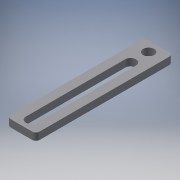
# Autodesk Inventor part: ButtonLockerV2
Saved by Autodesk Inventor 2018 (Build 220112000, 112)
## iProperties
Created: 2018-05-22
Part Number: ButtonLockerV2
Material: Generic
Document SubType Name: Modeling
Designer: reide
Density: 1 g/cm^3
Appearance: Default
Author: reide
Autodesk Inventor part; units mm, degrees
ref_plane "YZ Plane" through (0, 0, 0) normal (1, 0, 0) x (0, 1, 0)
ref_plane "XZ Plane" through (0, 0, 0) normal (0, 1, 0) x (-1, 0, 0)
ref_plane "XY Plane" through (0, 0, 0) normal (0, 0, 1) x (1, 0, 0)
sketch "Sketch1" plane through (0, 0, 0) normal (0, 0, 1) x (1, 0, 0)
  line L0 (35.2961, 108.9853) -> (93.2961, 108.9853)
  line L1 (35.2961, 103.4853) -> (35.2961, 108.9853)
  line L2 (93.2961, 103.4853) -> (35.2961, 103.4853)
  line L3 (93.2961, 108.9853) -> (93.2961, 103.4853)
  line L4 (2, 88) -> (126.0922, 88)
  line L5 (2, 80) -> (2, 88)
  line L6 (2, 80) -> (126.0922, 80)
  line L7 (126.0922, 80) -> (126.0922, 88)
  line L8 (11.7071, 1) -> (2, 1)
  line L9 (11.7071, 80) -> (11.7071, 1)
  line L10 (2, 80) -> (11.7071, 80)
  line L11 (2, 1) -> (2, 80)
  line L12 (126.0922, 80) -> (126.0922, 1)
  line L13 (126.0922, 1) -> (116.3851, 1)
  line L14 (126.0922, 80) -> (126.0922, 1)
  line L15 (116.3851, 80) -> (126.0922, 80)
  line L16 (116.3851, 1) -> (116.3851, 80)
  line L17 (102.7961, 70.9853) -> (96.2961, 70.9853)
  line L18 (102.7961, 108.9853) -> (102.7961, 70.9853)
  line L19 (95.2961, 108.9853) -> (102.7961, 108.9853)
  line L20 (95.2961, 103.4853) -> (95.2961, 108.9853)
  line L21 (96.2961, 103.4853) -> (95.2961, 103.4853)
  line L22 (96.2961, 103.4853) -> (96.2961, 70.9853)
  line L23 (32.2961, 70.9853) -> (25.7961, 70.9853)
  line L24 (32.2961, 103.4853) -> (32.2961, 70.9853)
  line L25 (33.2961, 103.4853) -> (32.2961, 103.4853)
  line L26 (33.2961, 108.9853) -> (33.2961, 103.4853)
  line L27 (25.7961, 108.9853) -> (33.2961, 108.9853)
  line L28 (25.7961, 70.9853) -> (25.7961, 108.9853)
  line L29 (64.2961, 108.9853) -> (64.2961, 70.9853)
  line L30 (64.2961, 108.9853) -> (68.2961, 108.9853)
  line L31 (68.2961, 108.9853) -> (60.2961, 108.9853)
  line L32 (60.2961, 108.9853) -> (66.2961, 108.9853)
  line L33 (66.2961, 70.4263) -> (60.2961, 70.4263)
  line L34 (60.2961, 70.4263) -> (60.2961, 108.9853)
  circle A0 centre (64.2961, 106.2353) radius 1.75
  line L35 (68.2961, 108.9853) -> (60.2961, 108.9853)
  line L36 (60.2961, 108.9853) -> (60.2961, 70.4263)
  line L37 (60.2961, 70.4263) -> (68.2961, 70.4263)
  line L38 (68.2961, 70.4263) -> (68.2961, 108.9853)
  line L39 (64.2961, 106.2353) -> (64.2961, 101.2353)
  line L40 (68.2961, 89.7058) -> (76.3965, 89.7058)
  arc A1 (62.5461, 73.1763) -> (66.0461, 73.1763) centre (64.2961, 73.1763) ccw
  line L41 (62.7961, 101.2353) -> (65.7961, 101.2353)
  circle A2 centre (64.2961, 106.2353) radius 1.6
  circle A3 centre (64.2961, 101.2353) radius 1.75
  line L42 (62.5461, 73.1763) -> (66.0461, 73.1763)
  line L43 (66.0461, 73.1763) -> (66.0461, 101.2353)
  line L44 (66.0461, 101.2353) -> (62.5461, 101.2353)
  line L45 (62.5461, 101.2353) -> (62.5461, 73.1763)
  circle A4 centre (64.2961, 84) radius 1.6
  point P0 (0, 0)
extrude "Extrusion1" add sketch "Sketch1" along normal blind 2 contours L0 L29 A0 L2 L34 | L0 L38 L2 L29 A0 | L2 L29 A3 L45 L4 L34 | L2 L38 L4 L43 A3 L29 | L4 L45 L6 L34 | L6 L45 A1 L43 L38 L37 L33 L34 | L38 L6 L43 L4
fillet "Fillet1" radius 1 4 edges at (60.2961, 108.9853, 1) (68.2961, 108.9853, 1) (60.2961, 70.4263, 1) (68.2961, 70.4263, 1)
body "Solid1"
